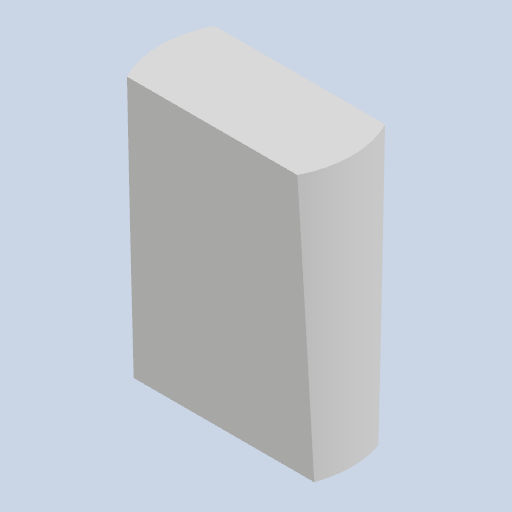
# Autodesk Inventor part: middle_gear_vtilka_shtift
Saved by Autodesk Inventor 2022 (Build 260153000, 153)
## iProperties
Created: 2024-12-03
Part Number: middle_gear_vtilka_shtift
Material: Типовые
Document SubType Name: Modeling
Designer: Andrey
Density: 1 g/cm^3
Appearance: По умолчанию
Author: Andrey
Autodesk Inventor part; units mm, degrees
ref_plane "YZ Plane" through (0, 0, 0) normal (1, 0, 0) x (0, 1, 0)
ref_plane "XZ Plane" through (0, 0, 0) normal (0, 1, 0) x (-1, 0, 0)
ref_plane "XY Plane" through (0, 0, 0) normal (0, 0, 1) x (1, 0, 0)
sketch "Эскиз1" plane through (0, 0, 0) normal (1, 0, 0) x (0, 1, 0)
  line L0 (4.2947, -1.2) -> (3.8947, -1.2) projected
  line L1 (3.8947, -1.2) -> (0, -1.2) projected
  line L2 (0, -1.2) -> (-1, -1.2) projected
  line L3 (-4, 22.6194) -> (-4, -13.7271) projected
  line L4 (-1, -1.2) -> (-2.2, -1.2) projected
  line L5 (-2.2, -2.95) -> (-2.2, -1.2) projected
  line L6 (-2.2504, -1.2) -> (-4.2, -1.2) projected
  line L7 (-2.2, -1.2) -> (-2.2504, -1.2) projected
  line L8 (-4.2947, 1.2) -> (4.2947, 1.2)
  line L9 (4.2947, 1.2) -> (4.2947, -1.2)
  line L10 (4.2947, -1.2) -> (-4.2947, -1.2)
  line L11 (-4.2947, -1.2) -> (-4.2947, 1.2)
  line L12 (-4.2947, 1.2) -> (4.2947, -1.2) construction
  line L13 (4.2947, 1.2) -> (-4.2947, -1.2) construction
  line L14 (4.2947, -1.35) -> (-4, -0.9878)
  line L15 (4.2947, -1.35) -> (4.2947, -1.2)
  line L16 (-4, -1.2) -> (-4, -0.9878)
  line L17 (4.2947, 0) -> (-4, 0)
  line L18 (4.2947, 1.35) -> (-4, 0.9878)
  line L19 (4.2947, 1.35) -> (4.2947, 1.2)
  point P0 (0, 0)
  point P1 (-4, 0.9878)
  dimension "d0" = 2.5
  dimension "d1" = 0.15
  constraints: 24 end point, 5 point on line, 3 midpoint, 2 parallel, 2 perpendicular, 2 symmetric about line, 1 collinear, 1 horizontal, 1 vertical
  measures "d0" angle of L1 L14
  measures "d1" distance of L14.start L0.start
extrude "Выдавливание1" add sketch "Эскиз1" along normal mid plane 6 contours L15 L14 L1 L0 | L0 L1 L14 L3 L17 L9 | L17 L3 L18 L8 L9 | L8 L18 L19
sketch "Эскиз2" plane through (-3, 4.2947, 1.35) normal (0, 1, 0) x (1, 0, 0)
  line L0 (5.25, 0.15) -> (0.75, 0.15) projected
  arc A0 (0.75, 0.15) -> (5.25, 0.15) centre (3, 1.35) ccw projected
  line L1 (0.75, 2.55) -> (5.25, 2.55) projected
  arc A1 (5.25, 2.55) -> (0.75, 2.55) centre (3, 1.35) ccw projected
  circle A2 centre (3, 1.35) radius 2.55
  line L2 (0, 0) -> (6, 0) projected
  line L3 (6, 2.7) -> (6, 0) projected
  line L4 (0, 2.7) -> (6, 2.7) projected
  line L5 (0, 0) -> (0, 2.7) projected
  arc A3 (5.6949, 2.55) -> (0.3051, 2.55) centre (3, 1.35) ccw projected
  arc A4 (0.3051, 0.15) -> (5.6949, 0.15) centre (3, 1.35) ccw projected
  circle A5 centre (3, 1.35) radius 2.95
  point P0 (3, 1.35)
  point P1 (0.8367, 0)
  point P2 (0.8367, 2.7)
  point P3 (5.1633, 2.7)
  point P4 (5.1633, 0)
  point P5 (5.623, 2.7)
  point P6 (5.6949, 0.15)
  point P7 (5.623, 0)
  point P8 (0.377, 0)
  point P9 (0.3051, 0.15)
  point P10 (0.3051, 2.55)
  point P11 (0.377, 2.7)
  constraints: 2 coincident, 6 other
extrude "Выдавливание2" cut sketch "Эскиз2" against normal blind 10 contours A4 A5 A3 L4 L3 L2 | L2 L5 L4 A3 A5 A4
